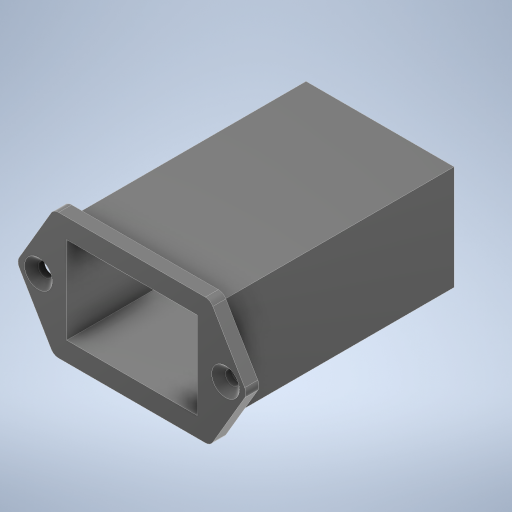
# Autodesk Inventor part: BatteryHolder_DigiKEY
Saved by Autodesk Inventor 2023 (Build 270158000, 158)
## iProperties
Created: 2022-10-05
Part Number: BatteryHolder_DigiKEY
Material: ABS Plastic
Document SubType Name: Modeling
Designer: jeanp
Density: 1.06 g/cm^3
Appearance: Smooth - Black
Author: jeanp
Autodesk Inventor part; units mm, degrees
ref_plane "YZ Plane" through (0, 0, 0) normal (1, 0, 0) x (0, 1, 0)
ref_plane "XZ Plane" through (0, 0, 0) normal (0, 1, 0) x (-1, 0, 0)
ref_plane "XY Plane" through (0, 0, 0) normal (0, 0, 1) x (1, 0, 0)
sketch "Sketch1" plane through (0, 0, 0) normal (0, 0, 1) x (1, 0, 0)
  line L0 (-25.9071, 1.0114) -> (-18.5795, 13.5114)
  line L1 (-16.8541, 14.5) -> (16.8541, 14.5)
  line L2 (18.5795, 13.5114) -> (25.9071, 1.0114)
  arc A0 (-16.8541, 14.5) -> (-18.5795, 13.5114) centre (-16.8541, 12.5) ccw
  arc A1 (18.5795, 13.5114) -> (16.8541, 14.5) centre (16.8541, 12.5) ccw
  line L3 (-28.1394, 0) -> (29.237, 0) construction
  line L4 (-25.9071, -1.0114) -> (-18.5795, -13.5114)
  line L5 (-16.8541, -14.5) -> (16.8541, -14.5)
  line L6 (18.5795, -13.5114) -> (25.9071, -1.0114)
  arc A2 (-18.5795, -13.5114) -> (-16.8541, -14.5) centre (-16.8541, -12.5) ccw
  arc A3 (16.8541, -14.5) -> (18.5795, -13.5114) centre (16.8541, -12.5) ccw
  arc A4 (-25.9071, 1.0114) -> (-25.9071, -1.0114) centre (-24.1817, 0) ccw
  arc A5 (25.9071, -1.0114) -> (25.9071, 1.0114) centre (24.1817, 0) ccw
  point P0 (0, 0)
  point P1 (-26.5, 0)
  point P2 (-18, 14.5)
  point P3 (18, 14.5)
  point P4 (26.5, 0)
  point P5 (-18, -14.5)
  point P6 (18, -14.5)
  dimension "d0" = 53
  dimension "d1" = 26.5
  dimension "d2" = 14.5
  dimension "d3" = 36
  dimension "d4" = 18
  dimension "d5" = 2
  dimension "d6" = 2
  constraints: 14 end point, 12 point on circle, 12 point on line, 8 symmetric about line, 8 tangent, 6 centre point, 3 horizontal, 2 equal radius, 2 other
  measures "d0" distance of point (26.5, 0) point (-26.5, 0)
  measures "d1" distance of point (0, 0) point (26.5, 0)
  measures "d2" distance from line of L1 point (0, 0)
  measures "d3" distance of point (-18, 14.5) point (18, 14.5)
  measures "d4" horizontal distance of point (0, 0) point (18, 14.5)
  measures "d5" radius of A0
  measures "d6" radius of A4
extrude "Extrusion1" add sketch "Sketch1" against normal blind 3
sketch "Sketch2" plane through (0, 0, 0) normal (0, 0, 1) x (1, 0, 0)
  point P0 (0, 0)
  point P1 (-21.5, 0)
  point P2 (21.5, 0)
  dimension "d9" = 43
  dimension "d10" = 21.5
  measures "d9" distance of point (-21.5, 0) point (21.5, 0)
  measures "d10" distance of point (21.5, 0) point (0, 0)
hole "Hole1" at (-21.5, 0, 0) at (21.5, 0, 0) direction (0, 0, -1) diameter 3.2 end through all countersink diameter 6.35 countersink angle 90 clearance for "Flat Head Machine Screw" size "M3" standard "Ansi Metric M Profile"
sketch "Sketch3" plane through (0, 0, -3) normal (0, 0, -1) x (-1, 0, 0)
  line L0 (-17, 12) -> (17, 12)
  line L1 (17, 12) -> (17, -12)
  line L2 (17, -12) -> (-17, -12)
  line L3 (-17, -12) -> (-17, 12)
  point P0 (0, 0)
  dimension "d18" = 24
  dimension "d19" = 34
  dimension "d20" = 17
  dimension "d21" = 12
  constraints: 8 end point, 2 parallel, 1 horizontal, 1 perpendicular
  measures "d18" distance of L2.end L0.start
  measures "d19" distance of L0.start L0.end
  measures "d20" distance from line of L1 point (0, 0)
  measures "d21" distance from line of point (0, 0) L2
extrude "Extrusion2" add sketch "Sketch3" along normal blind 54
sketch "Sketch4" plane through (0, 0, 0) normal (0, 0, 1) x (1, 0, 0)
  line L0 (-15, 10) -> (15, 10)
  line L1 (15, 10) -> (15, -10)
  line L2 (15, -10) -> (-15, -10)
  line L3 (-15, -10) -> (-15, 10)
  point P0 (0, 0)
  dimension "d24" = 30
  dimension "d25" = 20
  dimension "d26" = 15
  dimension "d27" = 10
  constraints: 8 end point, 2 parallel, 1 horizontal, 1 perpendicular
  measures "d24" distance of L0.start L0.end
  measures "d25" distance of L0.end L1.end
  measures "d26" distance from line of point (0, 0) L1
  measures "d27" distance from line of L0 point (0, 0)
extrude "Extrusion3" cut sketch "Sketch4" against normal blind 49
equation "\"d1\" = 0.5 * d0"
equation "\"d4\" = 0.5 * d3"
equation "\"d10\" = 0.5 * d9"
equation "\"d20\" = 0.5 * d19"
equation "\"d21\" = 0.5 * d18"
equation "\"d26\" = 0.5 * d24"
equation "\"d27\" = 0.5 * d25"
body "Solid1"
